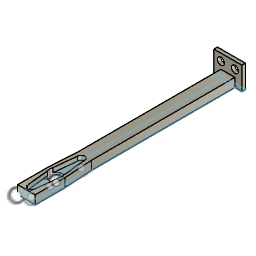
MG92B Tameron Servo Arm v3 (Autodesk Fusion 360 design; units mm, degrees)
Autodesk Fusion 360 part; units mm, degrees
sketch "arm sketch" plane through (0, 0, 0) normal (0, 0, 1) x (1, 0, 0)
  circle A0 centre (-0.0034, 0.0021) radius 3.65
  arc A1 (-0.0006, -3.625) -> (0, -3.625) centre (0, 0) ccw
  line L0 (0, -3.625) -> (0, -3.6479)
  line L1 (0, -3.625) -> (0, -3.6479)
  line L2 (1.986, 14.5075) -> (3.33, 1.4889)
  line L3 (-3.3369, 1.4889) -> (-2.0034, 14.2947)
  line L4 (-3.3369, -1.4847) -> (-1.9929, -14.5033)
  line L5 (1.9965, -14.3152) -> (3.3333, -1.4773)
  line L6 (-4.0034, 16.3021) -> (-5.0034, 0.0021)
  line L7 (3.9966, 16.3021) -> (4.9966, 0.0021)
  line L8 (4.9966, 0.0021) -> (4.9966, -16.9979)
  line L9 (-5.0034, -17.9979) -> (-5.0034, 0.0021)
  line L10 (4.9966, -16.9979) -> (-5.0034, -16.9979)
  line L11 (-0.0449, 98) -> (7.9551, 98.0037)
  line L12 (-0.0449, 98) -> (-8.0449, 97.9963)
  line L13 (-4.0034, 16.3021) -> (-4.0449, 97.9982)
  line L14 (3.9966, 16.3021) -> (3.9551, 98.0018)
  line L15 (-8.0449, 97.9963) -> (-8.0458, 99.9963)
  line L16 (-8.0458, 99.9963) -> (7.9542, 100.0044)
  line L17 (7.9542, 100.0044) -> (7.9551, 98.0037)
  arc A2 (-1.9929, -14.5033) -> (1.9965, -14.3152) centre (-0.0034, -14.2979) ccw
  arc A3 (1.986, 14.5075) -> (-2.0034, 14.2947) centre (-0.0034, 14.3021) ccw
  dimension "d13" = 7.3
  dimension "d30" = 14.3
  dimension "d31" = 14.3
  dimension "d32" = 4
  dimension "d33" = 4
  dimension "d50" = 5
  dimension "d52" = 5
  dimension "d55" = 1
  dimension "d69" = 98
  dimension "d71" = 8
  dimension "d72" = 8
  dimension "d73" = 2
  dimension "d74" = 16
  constraint coincident A0 L0.end
  constraint coincident A0 L2.end
  constraint tangent L2 A3
  constraint coincident A0 L3.start
  constraint coincident A0 L4.start
  constraint tangent L4 A2
  constraint parallel L2 L4
  constraint coincident A0 L5.end
  constraint parallel L3 L5
  constraint perpendicular L9 L10
  constraint midpoint L12 L13.end
  constraint midpoint L11 L14.end
  constraint perpendicular L12 L15
  constraint perpendicular L14 L16
  measures "d13" diameter of A0
  measures "d30" distance of A0.centre A3.centre
  measures "d31" distance of A0.centre A2.centre
  measures "d32" diameter of A2
  measures "d33" diameter of A3
  measures "d50" distance of A0.centre L6.end
  measures "d52" distance of A0.centre L7.end
  measures "d55" distance of L9.start L10.end
  measures "d69" distance of A1.centre L11.start
  measures "d71" distance of L11.start L11.end
  measures "d72" distance of L11.start L12.end
  measures "d73" distance of L12.end L15.end
  measures "d74" distance of L15.end L16.end
extrude "Extrude14" add sketch "arm sketch" along normal blind 2.5 contours A0 L2 L3 A3 | A0 L4 L5 A2 makes body 1 at (-0.0069, 10.8181, 0) makes body 2 at (0.0014, -10.8221, 0)
extrude "Extrude15" add sketch "arm sketch" along normal blind 5 contours L6 L7 L8 L9 L10 L11 L12 L13 L14 bodies 1 2
extrude "Extrude16" add sketch "arm sketch" along normal blind 13 contours L11 L12 L15 L16 L17 bodies 1
sketch "bolts" plane through (-0.0507, 100.0004, 0) normal (-0.000507, 1, 0) x (-1, -0.000507, 0)
  line L0 (-8.0049, 0) -> (7.9951, 0)
  line L1 (7.9951, 0) -> (7.9951, 13)
  line L2 (7.9951, 13) -> (-8.0049, 13)
  line L3 (-8.0049, 13) -> (-8.0049, 0)
  circle A0 centre (-4.0049, 9) radius 2
  circle A1 centre (3.9951, 9) radius 2
  dimension "d85" = 8
  dimension "d86" = 4
  dimension "d87" = 4
  measures "d85" distance of A0.centre A1.centre
  measures "d86" diameter of A0
  measures "d87" diameter of A1
extrude "Extrude17" cut sketch "bolts" against normal blind 5 contours A0 | A1 bodies 1
named bodies: "servo arm"
